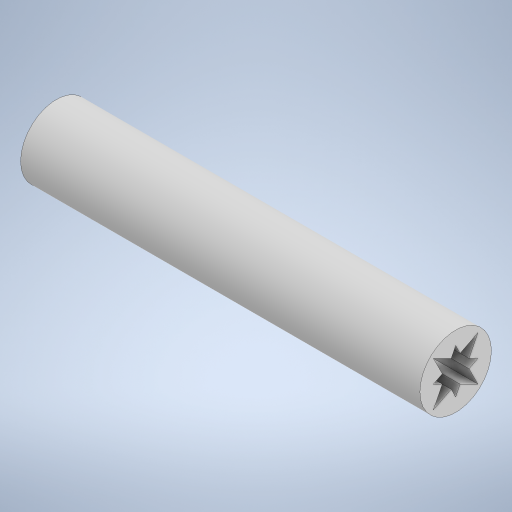
# Autodesk Inventor part: gear_shaft
Saved by Autodesk Inventor 2024 (Build 280153000, 153)
## iProperties
Created: 2023-05-17
Part Number: gear_shaft
Material: Generic
Document SubType Name: Modeling
Designer: chris
Density: 1 g/cm^3
Appearance: Default
Author: chris
Autodesk Inventor part; units mm, degrees
ref_plane "YZ Plane" through (0, 0, 0) normal (1, 0, 0) x (0, 1, 0)
ref_plane "XZ Plane" through (0, 0, 0) normal (0, 1, 0) x (-1, 0, 0)
ref_plane "XY Plane" through (0, 0, 0) normal (0, 0, 1) x (1, 0, 0)
sketch "Sketch1" plane through (0, 0, 0) normal (1, 0, 0) x (0, 1, 0)
  circle A0 centre (0, 0) radius 3.85
  dimension "d0" = 7.7
  constraints: 1 centre point, 1 coincident
  measures "d0" diameter of A0
extrude "Extrusion1" add sketch "Sketch1" along normal blind 5
sketch "Sketch2" plane through (5, 0, 0) normal (1, 0, 0) x (0, 0, -1)
  circle A0 centre (0, 0) radius 3.85
  dimension "d3" = 7.7
  constraints: 1 centre point, 1 coincident
  measures "d3" diameter of A0
extrude "Extrusion2" add sketch "Sketch2" along normal blind 18.5
sketch "Sketch5" plane through (0, 0, 0) normal (-1, 0, 0) x (0, 0, 1)
  circle A0 centre (0, 0) radius 2.4
  line L0 (0, 0) -> (-2.4, 0)
  line L1 (-2.4, 0) -> (-2.4, 2.4)
  line L2 (-2.4, 2.4) -> (0, 2.4)
  line L3 (0, 2.4) -> (0, 0)
  line L4 (-2.4, 2.4) -> (2.4, 2.4)
  line L5 (2.4, 2.4) -> (2.4, -2.4)
  line L6 (2.4, -2.4) -> (-2.4, -2.4)
  line L7 (-2.4, -2.4) -> (-2.4, 2.4)
  line L8 (-2.4, 2.4) -> (2.4, 0)
  line L9 (-2.4, -2.4) -> (2.4, 0)
  line L10 (-2.4, 0) -> (2.4, 2.4)
  line L11 (-2.4, 0) -> (2.4, -2.4)
  line L12 (0, 2.4) -> (2.4, -2.4)
  line L13 (-2.4, -2.4) -> (0, 2.4)
  line L14 (-2.4, 2.4) -> (0, -2.4)
  line L15 (0, -2.4) -> (2.4, 2.4)
  point P0 (1.44, -0.48)
  point P1 (1.44, 0.48)
  point P2 (0.48, 1.44)
  point P3 (-0.48, 1.44)
  point P4 (-1.44, 0.48)
  point P5 (-1.44, -0.48)
  point P6 (-0.48, -1.44)
  point P7 (0.48, -1.44)
  dimension "d23" = 4.8
  constraints: 32 end point, 5 parallel, 4 perpendicular, 2 horizontal, 2 midpoint, 1 centre point, 1 coincident
  measures "d23" diameter of A0
extrude "Extrusion5" cut sketch "Sketch5" against normal blind 10 contours L9 L12 L15 L8 | L15 L8 L12 L10 A0 | A0 L10 L15 | L12 L11 A0 | A0 L11 L15 L9 L12 | L15 L12 L8 | L9 L15 L12 | L12 L10 L3 | L3 L8 L13 | L14 L9 L11 L15 | L12 L15 L9 L11 L14 L0 L3 L8 | L8 L10 L12 | L15 L11 L9 | L8 L13 L10 L14 A0 | A0 L14 L8 | L10 L13 L8 | L3 L0 L13 L10 | L9 L13 A0 | A0 L13 L11 L14 L9 | L14 L11 L9 | L10 L14 L0 | L0 L13 L11 | L13 L14 L10 | L11 L13 L14
sketch "Sketch7" plane through (0, 0, 0) normal (-1, 0, 0) x (0, 0, 1)
  circle A0 centre (0, 0) radius 3.85
  constraints: 1 centre point, 1 coincident
extrude "Extrusion7" cut sketch "Sketch7" against normal blind 2
mirror "Mirror1" about plane through (23.5, 0, 0) normal (1, 0, 0)
body "Solid1"
